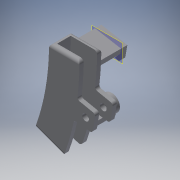
# Autodesk Inventor part: Frame Holder
Saved by Autodesk Inventor 2018.3 (Build 223284000, 284)
## iProperties
Created: 2020-12-21
Material: Generic
Vendor: HHMI: JRC - ID&F
Document SubType Name: Modeling
Designer: winnubstj
Density: 1 g/cm^3
Appearance: Default
AfterDocSave0: file://Part Number Cleaner
Author: winnubstj
Revision Number: 0
Autodesk Inventor part; units mm, degrees
sketch "Outer Wall" plane through (0, 0, 0) normal (0, 0, 1) x (1, 0, 0)
  arc A0 (211.3626, -76.527) -> (224.79, 0) centre (0, 0) ccw
  line L0 (224.79, 0) -> (254, 0)
  line L1 (211.3626, -76.527) -> (238.8111, -86.5174)
  line L2 (-53.8883, 0) -> (323.3301, 0) projected
  arc A1 (266.7706, -51.2851) -> (268.8758, -38.762) centre (0, 0) ccw
  line L3 (263.9447, -53.3238) -> (251.0915, -51.6317)
  line L4 (266.8719, -35.9113) -> (254.1719, -33.3077)
  circle A2 centre (259.899, -43.6914) radius 2.667
  arc A3 (252.1604, -30.5143) -> (254, 0) centre (0, 0) ccw
  arc A4 (238.8111, -86.5174) -> (248.2772, -53.6138) centre (0, 0) ccw
  arc A5 (252.1604, -30.5143) -> (254.1719, -33.3077) centre (254.682, -30.8195) ccw
  arc A6 (251.0915, -51.6317) -> (248.2772, -53.6138) centre (250.76, -54.1499) ccw
  arc A7 (268.8758, -38.762) -> (266.8719, -35.9113) centre (266.3618, -38.3995) ccw
  arc A8 (263.9447, -53.3238) -> (266.7706, -51.2851) centre (264.2762, -50.8056) ccw
  line L5 (252.6208, -32.3037) -> (265.7624, -52.8654)
  line L6 (268.4398, -36.9388) -> (249.2974, -52.0733)
  arc A9 (214.9429, -77.8301) -> (228.6, 0) centre (0, 0) ccw
  line L7 (0, 0) -> (240.03, -42.3238)
  arc A10 (225.0869, -81.5222) -> (239.395, 0) centre (0, 0) ccw
  point P0 (266.3081, -53.635)
  point P1 (269.2071, -36.39)
  point P2 (235.7908, -41.3841)
  dimension "d9" = 29.21
  dimension "d25" = 7.5
  dimension "d28" = 12.7
  dimension "d36" = 5.334
  dimension "d45" = 2.54
  dimension "d46" = 2.54
  dimension "d47" = 12.7
  dimension "d48" = 3.81
  dimension "d92" = 254
  dimension "d118" = 240.03
  dimension "d119" = 10
  dimension "d252" = 20
  constraints: 27 point on circle, 14 end point, 11 centre point, 8 coincident, 8 tangent, 7 point on line, 3 equal radius, 2 horizontal alignment, 1 equal length, 1 midpoint
  measures "d9" distance of L0.start L0.end
  measures "d25" angle of L3 L2
  measures "d36" diameter of A2
  measures "d45" radius of A5
  measures "d46" radius of A7
  measures "d47" horizontal distance of L4.start L4.end
  measures "d48" radial gap between concentric circles of A9 A0
  measures "d92" radius of A3
  measures "d118" horizontal distance of L7.start L7.end
  measures "d119" angle of L7 L2
  measures "d252" angle of L2 L1
extrude "Extrusion2" add sketch "Outer Wall" along normal blind 4 contours A0 L7 A9 L1 | A0 L0 A9 L7 | A9 L7 A10 L1 | A9 L0 A10 L7 | A10 L0 A3 A5 L5 A2 L6 A6 A4 L1 | L6 A2 L5 A8 L3 A6 | L6 L5 A2 | A2 L5 L6 | A5 L4 A7 L6 A2 L5 | A2 L6 L5 | L5 L6 A2 | A2 L6 A7 A1 A8 L5
hole "Hole2" at (259.899, -43.6914, 0) direction (0, 0, 1) diameter 6.35 depth 25.4
extrude "Extrusion3" add sketch "Outer Wall" against normal blind 12.954 contours A0 L7 A9 L1 | A0 L0 A9 L7
ref_plane "Mirror Plane" through (0, 0, -6.477) normal (0, 0, -1) x (-1, 0, 0)
mirror "Mirror1" about plane through (0, 0, -6.477) normal (0, 0, -1) of "Extrusion2", "Hole2"
fillet "Fillet2" radius 3.175 9 edges at (254, 0, 2) (238.8111, -86.5174, 2) (224.79, 0, -6.477) (238.8111, -86.5174, -14.954) (254, 0, -14.954) (239.395, 0, -16.954) (225.0869, -81.5222, -16.954) (225.0869, -81.5222, 4) (239.395, 0, 4)
ref_plane "Mounting Plane" through (253.9799, -3.175, -16.954) normal (0, 0, -1) x (-1, 0, 0)
sketch "Back Nut Holder" plane through (253.9799, -3.175, -16.954) normal (0, 0, -1) x (-1, 0, 0)
  circle A0 centre (-5.9191, -40.5164) radius 3.175 projected
  line L0 (-4.0953, -35.0385) -> (-0.2632, -39.3569)
  line L1 (-0.2632, -39.3569) -> (-2.087, -44.8348)
  line L2 (-2.087, -44.8348) -> (-7.7429, -45.9943)
  line L3 (-7.7429, -45.9943) -> (-11.575, -41.6759)
  line L4 (-11.575, -41.6759) -> (-9.7512, -36.198)
  line L5 (-9.7512, -36.198) -> (-4.0953, -35.0385)
  line L6 (-12.892, -32.7363) -> (-0.192, -30.1327) projected
  circle A1 centre (-5.9191, -40.5164) radius 8.048
  point P0 (253.9799, 3.175)
  dimension "d202" = 10
  dimension "d203" = 3.048
  constraints: 12 end point, 2 coincident, 1 centre point, 1 parallel, 13 other
  measures "d202" distance between parallel lines of L2 L5
  measures "d203" distance edge to line of A1 L0
extrude "Extrusion9" add sketch "Back Nut Holder" along normal blind 4 contours A1
sketch "Mounting connectors" plane through (253.9799, -3.175, -16.954) normal (0, 0, -1) x (-1, 0, 0)
  line L0 (2.8226, -13.1866) -> (27.8226, -8.7784)
  line L1 (27.8226, -8.7784) -> (26.9543, -3.8544)
  line L2 (26.9543, -3.8544) -> (1.9543, -8.2625)
  line L3 (1.9543, -8.2625) -> (2.8226, -13.1866)
  line L4 (0, 0) -> (29.2123, 0) projected
  line L5 (12.3732, -67.351) -> (37.3732, -62.9428)
  line L6 (37.3732, -62.9428) -> (38.2415, -67.8669)
  line L7 (38.2415, -67.8669) -> (13.2415, -72.275)
  line L8 (13.2415, -72.275) -> (12.3732, -67.351)
  line L9 (14.1063, -80.3503) -> (41.5574, -70.3589) projected
  line L10 (29.2123, 0) -> (0, 0) projected
  line L11 (0.0003, -0.0402) -> (29.2123, 0)
  arc A0 (5.7027, -50.4388) -> (14.0912, -80.308) centre (253.9799, 3.175) ccw projected
  line L12 (24.8732, -65.1469) -> (15.3226, -10.9825)
  line L13 (253.9799, 3.175) -> (13.9499, -39.1488) projected
  arc A1 (29.2123, 0) -> (41.5574, -70.3589) centre (253.9799, 3.175) ccw projected
  point P0 (18.1891, -38.2091)
  point P1 (20.0979, -38.0647)
  dimension "d217" = 5
  dimension "d218" = 25
  dimension "d219" = 55
  dimension "d254" = 237.49
  constraints: 20 end point, 5 parallel, 3 midpoint, 3 perpendicular, 2 equal length, 1 collinear, 1 point on line
  measures "d217" distance of L2.end L0.start
  measures "d218" horizontal distance of L0.start L0.end
  measures "d219" distance between parallel lines of L5 L0
  measures "d254" distance from line of point (253.98, 3.175) L12
extrude "Extrusion11" add sketch "Mounting connectors" along normal blind 27
ref_plane "Work Plane10" through (253.9799, -3.175, -37.954) normal (0, 0, -1) x (-1, 0, 0)
sketch "holder platform" plane through (253.9799, -3.175, -37.954) normal (0, 0, -1) x (-1, 0, 0)
  line L0 (26.9543, -3.8544) -> (1.9543, -8.2625) projected
  line L1 (13.2415, -72.275) -> (38.2415, -67.8669) projected
  line L2 (26.9543, -3.8544) -> (27.8226, -8.7784) projected
  line L3 (26.9543, -3.8544) -> (1.9543, -8.2625)
  line L4 (1.9543, -8.2625) -> (3.9513, -19.5878)
  line L5 (3.9513, -19.5878) -> (28.9513, -15.1797)
  line L6 (28.9513, -15.1797) -> (26.9543, -3.8544)
  line L7 (12.3732, -67.351) -> (13.2415, -72.275) projected
  line L8 (38.2415, -67.8669) -> (13.2415, -72.275)
  line L9 (13.2415, -72.275) -> (11.2445, -60.9498)
  line L10 (11.2445, -60.9498) -> (36.2445, -56.5416)
  line L11 (36.2445, -56.5416) -> (38.2415, -67.8669)
  point P0 (253.9799, 3.175)
  dimension "d223" = 42
  constraints: 16 end point, 5 equal length, 3 perpendicular, 1 collinear
  measures "d223" distance between parallel lines of L10 L5
extrude "Extrusion12" add sketch "holder platform" along normal blind 6
ref_plane "Work Plane11" through (253.9799, -3.175, -37.954) normal (0, 0, -1) x (-1, 0, 0)
sketch "Screw holes" plane through (253.9799, -3.175, -37.954) normal (0, 0, -1) x (-1, 0, 0)
  line L0 (3.9513, -19.5878) -> (28.9513, -15.1797) projected
  line L1 (1.9543, -8.2625) -> (3.9513, -19.5878) projected
  line L2 (28.9513, -15.1797) -> (26.9543, -3.8544) projected
  line L3 (11.2445, -60.9498) -> (13.2415, -72.275) projected
  line L4 (36.2445, -56.5416) -> (11.2445, -60.9498) projected
  line L5 (38.2415, -67.8669) -> (36.2445, -56.5416) projected
  circle A0 centre (10.9161, -14.9375) radius 2.5
  circle A1 centre (29.2798, -61.1919) radius 2.5
  line L6 (19.3798, -62.9375) -> (10.9161, -14.9375)
  line L7 (10.9161, -14.9375) -> (20.8161, -13.1919)
  line L8 (20.8161, -13.1919) -> (29.2798, -61.1919)
  line L9 (29.2798, -61.1919) -> (19.3798, -62.9375)
  line L10 (23.7445, -58.7457) -> (16.4513, -17.3837)
  line L11 (29.2798, -61.1919) -> (10.9161, -14.9375)
  line L12 (19.3798, -62.9375) -> (20.8161, -13.1919)
  line L13 (12.792, -9.7835) -> (16.3176, -13.9851)
  line L14 (16.3176, -13.9851) -> (14.4416, -19.1391)
  line L15 (14.4416, -19.1391) -> (9.0401, -20.0916)
  line L16 (9.0401, -20.0916) -> (5.5146, -15.89)
  line L17 (5.5146, -15.89) -> (7.3905, -10.7359)
  line L18 (7.3905, -10.7359) -> (12.792, -9.7835)
  line L19 (27.8226, -8.7784) -> (2.8226, -13.1866) projected
  line L20 (27.331, -66.3188) -> (23.8653, -62.0676)
  line L21 (23.8653, -62.0676) -> (25.8141, -56.9407)
  line L22 (25.8141, -56.9407) -> (31.2286, -56.0649)
  line L23 (31.2286, -56.0649) -> (34.6942, -60.3161)
  line L24 (34.6942, -60.3161) -> (32.7454, -65.4431)
  line L25 (32.7454, -65.4431) -> (27.331, -66.3188)
  point P0 (253.9799, 3.175)
  point P1 (20.0979, -38.0647)
  point P2 (20.0979, -38.0647)
  point P3 (20.5863, -12.961)
  dimension "d227" = 5
  dimension "d228" = 9.9
  dimension "d229" = 48
  dimension "d231" = 9.5
  constraints: 38 end point, 5 coincident, 5 midpoint, 4 parallel, 2 centre point, 1 equal length, 1 equal radius, 1 perpendicular, 26 other
  measures "d227" diameter of A0
  measures "d228" horizontal distance of L6.end L7.end
  measures "d229" vertical distance of L6.start L6.end
  measures "d231" distance between parallel lines of L18 L15
extrude "Extrusion13" cut sketch "Screw holes" along normal blind 4 contours L16 L17 L19 L13 L7 A0 L6 L0 | L0 L6 L15 L16 | L6 A0 L11 L0 | L0 L11 L15 L6 | L17 L18 L13 L19 | L11 A0 L7 L14 L0 | L0 L14 L15 L11 | L22 L8 L4 L11 | L11 L4 L21 L22 | L20 L21 L4 L11 A1 L9 | L9 A1 L8 L4 L23 L24 L25 L20 | L4 L8 A1 L11 | L22 L23 L4 L8
hole "Hole13" at (243.0638, -18.1125, -37.954) direction (0, 0, -1) diameter 5 depth 25.4 tip angle 118
hole "Hole14" at (224.7001, -64.3669, -37.954) direction (0, 0, -1) diameter 5 depth 25.4 tip angle 118
body "Solid2"
